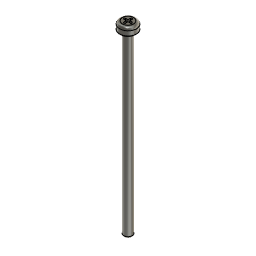
MG996R_Screw v2 (Autodesk Fusion 360 design; units mm, degrees)
Autodesk Fusion 360 part; units mm, degrees
sketch "Sketch1" plane through (0, 0, 0) normal (0, 0, 1) x (1, 0, 0)
  circle A0 centre (0, 0) radius 0.75
  dimension "d1" = 1.5
  constraint coincident A0.centre origin
  measures "d1" diameter of A0
extrude "Extrude1" add sketch "Sketch1" along normal blind 33
sketch "Sketch2" plane through (0, 0, 33) normal (0, 0, 1) x (-1, 0, 0)
  circle A0 centre (0, 0) radius 0.75
  circle A1 centre (0, 0) radius 1.5
  dimension "d4" = 3
  constraint concentric A0 A1
  measures "d4" diameter of A1
extrude "Extrude2" add sketch "Sketch2" against normal blind 1.5
fillet "Fillet1" radius 0.5 1 edges at (1.3985, 0.5424, 33)
fillet "Fillet2" radius 0.2 1 edges at (1.3985, -0.5424, 31.5)
sketch "Sketch3" plane through (0, 0, 33) normal (0, 0, 1) x (-1, 0, 0)
  circle A0 centre (0, 0) radius 1
  line L0 (0.6, 0.15) -> (-0.6, 0.15)
  arc A1 (-0.6, 0.15) -> (-0.6, -0.15) centre (-0.6, 0) ccw
  line L1 (-0.6, -0.15) -> (0.6, -0.15)
  arc A2 (0.6, -0.15) -> (0.6, 0.15) centre (0.6, 0) ccw
  line L2 (0.6, 0) -> (-0.6, 0) construction
  line L3 (-0.15, 0.6) -> (-0.15, -0.6)
  arc A3 (-0.15, -0.6) -> (0.15, -0.6) centre (0, -0.6) ccw
  line L4 (0.15, -0.6) -> (0.15, 0.6)
  arc A4 (0.15, 0.6) -> (-0.15, 0.6) centre (0, 0.6) ccw
  line L5 (0, 0.6) -> (0, -0.6) construction
  dimension "d11" = 0.3
  dimension "d12" = 1.2
  dimension "d13" = 0.3
  dimension "d14" = 1.2
  constraint tangent L0 A1
  constraint tangent A1 L1
  constraint parallel L0 L1
  constraint tangent L1 A2
  constraint tangent L0 A2
  constraint horizontal L2
  constraint coincident A0.centre origin
  constraint midpoint L2 A0.centre
  constraint tangent L3 A3
  constraint tangent A3 L4
  constraint parallel L3 L4
  constraint tangent L4 A4
  constraint tangent L3 A4
  constraint perpendicular L1 L5
  constraint midpoint L5 A0.centre
  measures "d11" distance of L0 L1
  measures "d12" distance of A1.end L1.end
  measures "d13" distance of L3 L4
  measures "d14" distance of A4.centre A3.centre
extrude "Extrude3" cut sketch "Sketch3" against normal blind 1.2 contours L0 L1 A2 L4 | L0 L1 L3 L4 | L0 L3 L4 A4 | L0 A1 L1 L3 | L1 L3 A3 L4
fillet "Fillet3" radius 0.3 1 edges at (-0.6992, -0.2712, 0)
